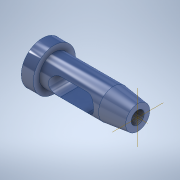
# Autodesk Inventor part: tool holder
Saved by Autodesk Inventor 2021.1 (Build 251245000, 245)
## iProperties
Created: 2021-02-18
Part Number: tool holder
Material: Generic
Document SubType Name: Modeling
Designer: Vamshi
Density: 1 g/cm^3
Appearance: Flaked Satin - Blue
Author: Vamshi
Autodesk Inventor part; units mm, degrees
ref_plane "YZ Plane" through (0, 0, 0) normal (1, 0, 0) x (0, 1, 0)
ref_plane "XZ Plane" through (0, 0, 0) normal (0, 1, 0) x (-1, 0, 0)
ref_plane "XY Plane" through (0, 0, 0) normal (0, 0, 1) x (1, 0, 0)
sketch "Sketch1" plane through (0, 0, 0) normal (0, 0, 1) x (1, 0, 0)
  line L0 (0, 0) -> (-95, 0)
  line L1 (-95, 0) -> (-95, 21)
  line L2 (-95, 21) -> (-83, 21)
  line L3 (-83, 21) -> (-83, 15)
  line L4 (-83, 15) -> (-24, 15)
  line L5 (-24, 15) -> (0, 12)
  line L6 (0, 12) -> (0, 0)
  dimension "d0" = 12
  dimension "d1" = 59
  dimension "d2" = 24
  dimension "d3" = 12
  dimension "d4" = 21
  dimension "d5" = 15
  constraints: 14 end point, 5 perpendicular, 1 horizontal
  measures "d0" distance of L1.end L2.end
  measures "d1" distance of L3.end L4.end
  measures "d2" horizontal distance of L4.end L5.end
  measures "d3" distance of L5.end L0.start
  measures "d4" distance of L0.end L1.end
  measures "d5" distance between parallel lines of L0 L4
revolve "Revolution1" add sketch "Sketch1" angle 360 about axis through (0, 0, 0) along (-1, 0, 0)
sketch "Sketch2" plane through (0, 0, 0) normal (0, 0, 1) x (1, 0, 0)
  line L0 (-65, 0) -> (-38, 0) construction
  line L1 (-65, -9) -> (-38, -9)
  line L2 (-38, 9) -> (-65, 9)
  arc A0 (-65, 9) -> (-65, -9) centre (-65, 0) ccw
  arc A1 (-38, -9) -> (-38, 9) centre (-38, 0) ccw
  line L3 (-95, -21) -> (-95, 21) projected
  point P0 (0, 0)
  point P1 (-51.5, 0)
  dimension "d7" = 27
  dimension "d8" = 30
  dimension "d9" = 9
  constraints: 8 end point, 4 point on circle, 4 tangent, 2 centre point, 1 horizontal, 1 midpoint, 1 parallel
  measures "d7" distance of L0.start L0.end
  measures "d8" distance from line of L3 L0.start
  measures "d9" radius of A0
extrude "Extrusion1" cut sketch "Sketch2" against normal through all both and the other way through all
sketch "Sketch3" plane through (0, 0, 0) normal (1, 0, 0) x (0, 0, -1)
  point P0 (0, 0)
  point P1 (0, 0)
  constraints: 1 coincident
hole "Hole1" at (0, 0, 0) direction (-1, 0, 0) diameter 12.9175 depth 40 tip angle 118 thread size "M14x1" class "6H" standard "ANSI Metric M Profile"
body "Solid1"
